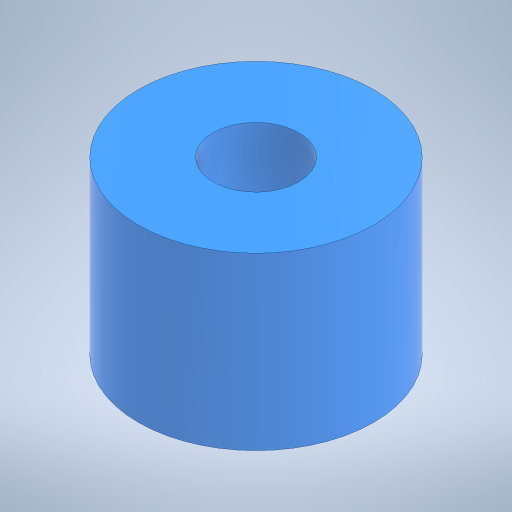
# Autodesk Inventor part: Claw_Bearing
Saved by Autodesk Inventor 2024 (Build 280153000, 153)
## iProperties
Created: 2023-10-18
Part Number: Claw_Bearing
Material: Generic
Document SubType Name: Modeling
Designer: tangl
Density: 1 g/cm^3
Appearance: Cyan
Author: tangl
Autodesk Inventor part; units mm, degrees
ref_plane "YZ Plane" through (0, 0, 0) normal (1, 0, 0) x (0, 1, 0)
ref_plane "XZ Plane" through (0, 0, 0) normal (0, 1, 0) x (-1, 0, 0)
ref_plane "XY Plane" through (0, 0, 0) normal (0, 0, 1) x (1, 0, 0)
sketch "Sketch1" plane through (0, 0, 0) normal (0, 1, 0) x (-1, 0, 0)
  circle A0 centre (0, 0) radius 8.7313
  circle A1 centre (0, 0) radius 3.175
  dimension "d0" = 17.4625
  dimension "d1" = 6.35
  constraints: 2 centre point, 2 coincident
  measures "d0" diameter of A0
  measures "d1" diameter of A1
extrude "Extrusion1" add sketch "Sketch1" along normal blind 12.7
body "Solid1"
